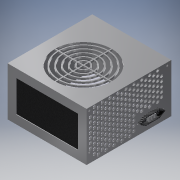
# Autodesk Inventor part: LC600H-12
Saved by Autodesk Inventor 2018.3 (Build 223284000, 284)
## iProperties
Created: 2019-03-04
Part Number: LC600H-12
Material: Generico
Document SubType Name: Modeling
Designer: AlfyPc
Density: 1 g/cm^3
Appearance: Alluminio - Scuro
Author: AlfyPc
Autodesk Inventor part; units mm, degrees
(part 1 of 4)
ref_plane "YZ Plane" through (0, 0, 0) normal (1, 0, 0) x (0, 1, 0)
ref_plane "XZ Plane" through (0, 0, 0) normal (0, 1, 0) x (-1, 0, 0)
ref_plane "XY Plane" through (0, 0, 0) normal (0, 0, 1) x (1, 0, 0)
sketch "Schizzo1" plane through (0, 0, 0) normal (0, 0, 1) x (1, 0, 0)
  line L0 (-70, 75) -> (70, 75)
  line L1 (70, 75) -> (70, -75)
  line L2 (70, -75) -> (-70, -75)
  line L3 (-70, -75) -> (-70, 75)
  line L4 (-70, 75) -> (70, -75) construction
  line L5 (70, 75) -> (-70, -75) construction
  line L6 (-70, 75) -> (70, 75) construction
  point P0 (0, 0)
  dimension "d0" = 140
  dimension "d1" = 0
  dimension "d2" = 150
  constraints: 14 end point, 2 horizontal, 2 midpoint, 2 parallel, 1 collinear, 1 perpendicular
  measures "d0" distance of L0.start L0.end
  measures "d1" distance between parallel lines of L0 L6
  measures "d2" distance of L0.end L1.end
extrude "Estrusione1" add sketch "Schizzo1" along normal blind 86
shell "Svuotamento1" thickness 3 removed faces 1 at (-23.3333, 25, 86)
sketch "Schizzo3" plane through (0, 0, 86) normal (0, 0, 1) x (1, 0, 0)
  line L0 (67, 72) -> (67, -72)
  line L1 (67, -72) -> (-67, -72)
  line L2 (-67, -72) -> (-67, 72)
  line L3 (-67, 72) -> (67, 72)
  line L4 (70, 75) -> (-70, 75)
  line L5 (-70, 75) -> (-70, -75)
  line L6 (-70, -75) -> (70, -75)
  line L7 (70, -75) -> (70, 75)
  line L8 (-1, 39.3407) -> (-1, 34.3396)
  line L9 (1, 34.3396) -> (1, 39.3407)
  line L10 (-1, 32.339) -> (-1, 25.837)
  line L11 (1, 25.837) -> (1, 32.339)
  line L12 (-1, 23.8362) -> (-1, 17.3328)
  line L13 (1, 17.3328) -> (1, 23.8362)
  line L14 (1, 0.3051) -> (1, 15.3314)
  line L15 (-1, 15.3314) -> (-1, 0.3051)
  line L16 (1, -28.1207) -> (1, -21.6038)
  line L17 (-1, -21.6038) -> (-1, -28.1207)
  line L18 (1, -36.6301) -> (1, -30.1237)
  line L19 (-1, -30.1237) -> (-1, -36.6301)
  line L20 (1, -45.1348) -> (1, -38.6315)
  line L21 (-1, -38.6315) -> (-1, -45.1348)
  line L22 (1, -60.6393) -> (1, -55.6382)
  line L23 (1, -53.6377) -> (1, -47.1356)
  line L24 (-1, -47.1356) -> (-1, -53.6377)
  line L25 (-1, -55.6382) -> (-1, -60.6393)
  line L26 (1, -19.5936) -> (1, -11.6493)
  line L27 (1, -9.6493) -> (1, -1.7051)
  line L28 (-1, -1.7051) -> (-1, -9.6493)
  line L29 (-1, -11.6493) -> (-1, -19.5936)
  line L30 (-8.9443, -9.6493) -> (-1, -9.6493)
  line L31 (-1, -11.6493) -> (-8.9443, -11.6493)
  line L32 (1, -9.6493) -> (8.9443, -9.6493)
  line L33 (8.9443, -11.6493) -> (1, -11.6493)
  line L34 (-17.4714, -9.6493) -> (-10.9545, -9.6493)
  line L35 (-10.9545, -11.6493) -> (-17.4714, -11.6493)
  line L36 (-49.99, -9.6493) -> (-27.9821, -9.6493)
  line L37 (-25.9808, -9.6493) -> (-19.4743, -9.6493)
  line L38 (-19.4743, -11.6493) -> (-25.9808, -11.6493)
  line L39 (-27.9821, -11.6493) -> (-49.99, -11.6493)
  line L40 (10.9545, -9.6493) -> (17.4714, -9.6493)
  line L41 (17.4714, -11.6493) -> (10.9545, -11.6493)
  arc A0 (1, -30.1237) -> (19.4743, -11.6493) centre (0, -10.6493) ccw
  arc A1 (19.4743, -9.6493) -> (1, 8.825) centre (0, -10.6493) ccw
  arc A2 (1, -28.1207) -> (17.4714, -11.6493) centre (0, -10.6493) ccw
  arc A3 (17.4714, -9.6493) -> (1, 6.8221) centre (0, -10.6493) ccw
  arc A4 (1, -21.6038) -> (10.9545, -11.6493) centre (0, -10.6493) ccw
  arc A5 (10.9545, -9.6493) -> (1, 0.3051) centre (0, -10.6493) ccw
  arc A6 (1, -19.5936) -> (8.9443, -11.6493) centre (0, -10.6493) ccw
  arc A7 (8.9443, -9.6493) -> (1, -1.7051) centre (0, -10.6493) ccw
  arc A8 (-1, -1.7051) -> (-8.9443, -9.6493) centre (0, -10.6493) ccw
  arc A9 (-8.9443, -11.6493) -> (-1, -19.5936) centre (0, -10.6493) ccw
  arc A10 (-1, 0.3051) -> (-10.9545, -9.6493) centre (0, -10.6493) ccw
  arc A11 (-10.9545, -11.6493) -> (-1, -21.6038) centre (0, -10.6493) ccw
  arc A12 (-1, 6.8221) -> (-17.4714, -9.6493) centre (0, -10.6493) ccw
  arc A13 (-17.4714, -11.6493) -> (-1, -28.1207) centre (0, -10.6493) ccw
  arc A14 (-1, 8.825) -> (-19.4743, -9.6493) centre (0, -10.6493) ccw
  arc A15 (-19.4743, -11.6493) -> (-1, -30.1237) centre (0, -10.6493) ccw
  arc A16 (-1, 15.3314) -> (-25.9808, -9.6493) centre (0, -10.6493) ccw
  arc A17 (-25.9808, -11.6493) -> (-1, -36.6301) centre (0, -10.6493) ccw
  arc A18 (-1, 17.3328) -> (-27.9821, -9.6493) centre (0, -10.6493) ccw
  arc A19 (-27.9821, -11.6493) -> (-1, -38.6315) centre (0, -10.6493) ccw
  arc A20 (-1, 23.8362) -> (-34.4855, -9.6493) centre (0, -10.6493) ccw
  arc A21 (-34.4855, -11.6493) -> (-1, -45.1348) centre (0, -10.6493) ccw
  arc A22 (-1, 25.837) -> (-36.4863, -9.6493) centre (0, -10.6493) ccw
  arc A23 (-36.4863, -11.6493) -> (-1, -47.1356) centre (0, -10.6493) ccw
  arc A24 (-1, 32.339) -> (-42.9884, -9.6493) centre (0, -10.6493) ccw
  arc A25 (-42.9884, -11.6493) -> (-1, -53.6377) centre (0, -10.6493) ccw
  arc A26 (-1, 34.3396) -> (-44.9889, -9.6493) centre (0, -10.6493) ccw
  arc A27 (-44.9889, -11.6493) -> (-1, -55.6382) centre (0, -10.6493) ccw
  arc A28 (-1, 39.3407) -> (-49.99, -9.6493) centre (0, -10.6493) ccw
  arc A29 (-49.99, -11.6493) -> (-1, -60.6393) centre (0, -10.6493) ccw
  arc A30 (1, -60.6393) -> (49.99, -11.6493) centre (0, -10.6493) ccw
  arc A31 (49.99, -9.6493) -> (1, 39.3407) centre (0, -10.6493) ccw
  arc A32 (1, -55.6382) -> (44.9889, -11.6493) centre (0, -10.6493) ccw
  arc A33 (44.9889, -9.6493) -> (1, 34.3396) centre (0, -10.6493) ccw
  arc A34 (1, -53.6377) -> (42.9884, -11.6493) centre (0, -10.6493) ccw
  arc A35 (42.9884, -9.6493) -> (1, 32.339) centre (0, -10.6493) ccw
  arc A36 (1, -47.1356) -> (36.4863, -11.6493) centre (0, -10.6493) ccw
  arc A37 (36.4863, -9.6493) -> (1, 25.837) centre (0, -10.6493) ccw
  arc A38 (1, -45.1348) -> (34.4855, -11.6493) centre (0, -10.6493) ccw
  arc A39 (34.4855, -9.6493) -> (1, 23.8362) centre (0, -10.6493) ccw
  arc A40 (1, -38.6315) -> (27.9821, -11.6493) centre (0, -10.6493) ccw
  arc A41 (27.9821, -9.6493) -> (1, 17.3328) centre (0, -10.6493) ccw
  arc A42 (1, -36.6301) -> (25.9808, -11.6493) centre (0, -10.6493) ccw
  arc A43 (25.9808, -9.6493) -> (1, 15.3314) centre (0, -10.6493) ccw
  line L42 (19.4743, -9.6493) -> (25.9808, -9.6493)
  line L43 (25.9808, -11.6493) -> (19.4743, -11.6493)
  line L44 (27.9821, -9.6493) -> (34.4855, -9.6493)
  line L45 (34.4855, -11.6493) -> (27.9821, -11.6493)
  line L46 (36.4863, -9.6493) -> (42.9884, -9.6493)
  line L47 (44.9889, -9.6493) -> (49.99, -9.6493)
  line L48 (49.99, -11.6493) -> (44.9889, -11.6493)
  line L49 (42.9884, -11.6493) -> (36.4863, -11.6493)
  point P0 (0, 0)
  constraints: 221 parallel, 84 end point, 12 point on line, 8 point on circle, 4 centre point, 121 other
extrude "Estrusione2" add sketch "Schizzo3" against normal blind 3 contours L0 L1 L2 L3
sketch "Schizzo4" plane through (70, -75, 0) normal (1, 0, 0) x (0, 0, -1)
  line L0 (-9, 7) -> (-7.5, 9.5981)
  line L1 (-7.5, 9.5981) -> (-4.5, 9.5981)
  line L2 (-4.5, 9.5981) -> (-3, 7)
  line L3 (-3, 7) -> (-4.5, 4.4019)
  line L4 (-4.5, 4.4019) -> (-7.5, 4.4019)
  line L5 (-7.5, 4.4019) -> (-9, 7)
  line L6 (-17, 7) -> (-15.5, 9.5981)
  line L7 (-15.5, 9.5981) -> (-12.5, 9.5981)
  line L8 (-12.5, 9.5981) -> (-11, 7)
  line L9 (-11, 7) -> (-12.5, 4.4019)
  line L10 (-12.5, 4.4019) -> (-15.5, 4.4019)
  line L11 (-15.5, 4.4019) -> (-17, 7)
  line L12 (-25, 7) -> (-23.5, 9.5981)
  line L13 (-23.5, 9.5981) -> (-20.5, 9.5981)
  line L14 (-20.5, 9.5981) -> (-19, 7)
  line L15 (-19, 7) -> (-20.5, 4.4019)
  line L16 (-20.5, 4.4019) -> (-23.5, 4.4019)
  line L17 (-23.5, 4.4019) -> (-25, 7)
  line L18 (-33, 7) -> (-31.5, 9.5981)
  line L19 (-31.5, 9.5981) -> (-28.5, 9.5981)
  line L20 (-28.5, 9.5981) -> (-27, 7)
  line L21 (-27, 7) -> (-28.5, 4.4019)
  line L22 (-28.5, 4.4019) -> (-31.5, 4.4019)
  line L23 (-31.5, 4.4019) -> (-33, 7)
  line L24 (-41, 7) -> (-39.5, 9.5981)
  line L25 (-39.5, 9.5981) -> (-36.5, 9.5981)
  line L26 (-36.5, 9.5981) -> (-35, 7)
  line L27 (-35, 7) -> (-36.5, 4.4019)
  line L28 (-36.5, 4.4019) -> (-39.5, 4.4019)
  line L29 (-39.5, 4.4019) -> (-41, 7)
  line L30 (-49, 7) -> (-47.5, 9.5981)
  line L31 (-47.5, 9.5981) -> (-44.5, 9.5981)
  line L32 (-44.5, 9.5981) -> (-43, 7)
  line L33 (-43, 7) -> (-44.5, 4.4019)
  line L34 (-44.5, 4.4019) -> (-47.5, 4.4019)
  line L35 (-47.5, 4.4019) -> (-49, 7)
  line L36 (-57, 7) -> (-55.5, 9.5981)
  line L37 (-55.5, 9.5981) -> (-52.5, 9.5981)
  line L38 (-52.5, 9.5981) -> (-51, 7)
  line L39 (-51, 7) -> (-52.5, 4.4019)
  line L40 (-52.5, 4.4019) -> (-55.5, 4.4019)
  line L41 (-55.5, 4.4019) -> (-57, 7)
  line L42 (-65, 7) -> (-63.5, 9.5981)
  line L43 (-63.5, 9.5981) -> (-60.5, 9.5981)
  line L44 (-60.5, 9.5981) -> (-59, 7)
  line L45 (-59, 7) -> (-60.5, 4.4019)
  line L46 (-60.5, 4.4019) -> (-63.5, 4.4019)
  line L47 (-63.5, 4.4019) -> (-65, 7)
  line L48 (-73, 7) -> (-71.5, 9.5981)
  line L49 (-71.5, 9.5981) -> (-68.5, 9.5981)
  line L50 (-68.5, 9.5981) -> (-67, 7)
  line L51 (-67, 7) -> (-68.5, 4.4019)
  line L52 (-68.5, 4.4019) -> (-71.5, 4.4019)
  line L53 (-71.5, 4.4019) -> (-73, 7)
  line L54 (-81, 7) -> (-79.5, 9.5981)
  line L55 (-79.5, 9.5981) -> (-76.5, 9.5981)
  line L56 (-76.5, 9.5981) -> (-75, 7)
  line L57 (-75, 7) -> (-76.5, 4.4019)
  line L58 (-76.5, 4.4019) -> (-79.5, 4.4019)
  line L59 (-79.5, 4.4019) -> (-81, 7)
  line L60 (-13, 13.9282) -> (-11.5, 16.5263)
  line L61 (-11.5, 16.5263) -> (-8.5, 16.5263)
  line L62 (-8.5, 16.5263) -> (-7, 13.9282)
  line L63 (-7, 13.9282) -> (-8.5, 11.3301)
  line L64 (-8.5, 11.3301) -> (-11.5, 11.3301)
  line L65 (-11.5, 11.3301) -> (-13, 13.9282)
  line L66 (-21, 13.9282) -> (-19.5, 16.5263)
  line L67 (-19.5, 16.5263) -> (-16.5, 16.5263)
  line L68 (-16.5, 16.5263) -> (-15, 13.9282)
  line L69 (-15, 13.9282) -> (-16.5, 11.3301)
  line L70 (-16.5, 11.3301) -> (-19.5, 11.3301)
  line L71 (-19.5, 11.3301) -> (-21, 13.9282)
  line L72 (-29, 13.9282) -> (-27.5, 16.5263)
  line L73 (-27.5, 16.5263) -> (-24.5, 16.5263)
  line L74 (-24.5, 16.5263) -> (-23, 13.9282)
  line L75 (-23, 13.9282) -> (-24.5, 11.3301)
  line L76 (-24.5, 11.3301) -> (-27.5, 11.3301)
  line L77 (-27.5, 11.3301) -> (-29, 13.9282)
  line L78 (-37, 13.9282) -> (-35.5, 16.5263)
  line L79 (-35.5, 16.5263) -> (-32.5, 16.5263)
  line L80 (-32.5, 16.5263) -> (-31, 13.9282)
  line L81 (-31, 13.9282) -> (-32.5, 11.3301)
  line L82 (-32.5, 11.3301) -> (-35.5, 11.3301)
  line L83 (-35.5, 11.3301) -> (-37, 13.9282)
  line L84 (-45, 13.9282) -> (-43.5, 16.5263)
  line L85 (-43.5, 16.5263) -> (-40.5, 16.5263)
  line L86 (-40.5, 16.5263) -> (-39, 13.9282)
  line L87 (-39, 13.9282) -> (-40.5, 11.3301)
  line L88 (-40.5, 11.3301) -> (-43.5, 11.3301)
  line L89 (-43.5, 11.3301) -> (-45, 13.9282)
  line L90 (-53, 13.9282) -> (-51.5, 16.5263)
  line L91 (-51.5, 16.5263) -> (-48.5, 16.5263)
  line L92 (-48.5, 16.5263) -> (-47, 13.9282)
  line L93 (-47, 13.9282) -> (-48.5, 11.3301)
  line L94 (-48.5, 11.3301) -> (-51.5, 11.3301)
  line L95 (-51.5, 11.3301) -> (-53, 13.9282)
  line L96 (-61, 13.9282) -> (-59.5, 16.5263)
  line L97 (-59.5, 16.5263) -> (-56.5, 16.5263)
  line L98 (-56.5, 16.5263) -> (-55, 13.9282)
  line L99 (-55, 13.9282) -> (-56.5, 11.3301)
  line L100 (-56.5, 11.3301) -> (-59.5, 11.3301)
  line L101 (-59.5, 11.3301) -> (-61, 13.9282)
  line L102 (-69, 13.9282) -> (-67.5, 16.5263)
  line L103 (-67.5, 16.5263) -> (-64.5, 16.5263)
  line L104 (-64.5, 16.5263) -> (-63, 13.9282)
  line L105 (-63, 13.9282) -> (-64.5, 11.3301)
  line L106 (-64.5, 11.3301) -> (-67.5, 11.3301)
  line L107 (-67.5, 11.3301) -> (-69, 13.9282)
  line L108 (-77, 13.9282) -> (-75.5, 16.5263)
  line L109 (-75.5, 16.5263) -> (-72.5, 16.5263)
  line L110 (-72.5, 16.5263) -> (-71, 13.9282)
  line L111 (-71, 13.9282) -> (-72.5, 11.3301)
  line L112 (-72.5, 11.3301) -> (-75.5, 11.3301)
  line L113 (-75.5, 11.3301) -> (-77, 13.9282)
  line L114 (-85, 13.9282) -> (-83.5, 16.5263)
  line L115 (-83.5, 16.5263) -> (-80.5, 16.5263)
  line L116 (-80.5, 16.5263) -> (-79, 13.9282)
  line L117 (-79, 13.9282) -> (-80.5, 11.3301)
  line L118 (-80.5, 11.3301) -> (-83.5, 11.3301)
  line L119 (-83.5, 11.3301) -> (-85, 13.9282)
  line L120 (-17, 20.8564) -> (-15.5, 23.4545)
  line L121 (-15.5, 23.4545) -> (-12.5, 23.4545)
  line L122 (-12.5, 23.4545) -> (-11, 20.8564)
  line L123 (-11, 20.8564) -> (-12.5, 18.2583)
  line L124 (-12.5, 18.2583) -> (-15.5, 18.2583)
  line L125 (-15.5, 18.2583) -> (-17, 20.8564)
  line L126 (-25, 20.8564) -> (-23.5, 23.4545)
  line L127 (-23.5, 23.4545) -> (-20.5, 23.4545)
  line L128 (-20.5, 23.4545) -> (-19, 20.8564)
  line L129 (-19, 20.8564) -> (-20.5, 18.2583)
  line L130 (-20.5, 18.2583) -> (-23.5, 18.2583)
  line L131 (-23.5, 18.2583) -> (-25, 20.8564)
  line L132 (-33, 20.8564) -> (-31.5, 23.4545)
  line L133 (-31.5, 23.4545) -> (-28.5, 23.4545)
  line L134 (-28.5, 23.4545) -> (-27, 20.8564)
  line L135 (-27, 20.8564) -> (-28.5, 18.2583)
  line L136 (-28.5, 18.2583) -> (-31.5, 18.2583)
  line L137 (-31.5, 18.2583) -> (-33, 20.8564)
  line L138 (-41, 20.8564) -> (-39.5, 23.4545)
  line L139 (-39.5, 23.4545) -> (-36.5, 23.4545)
  line L140 (-36.5, 23.4545) -> (-35, 20.8564)
  line L141 (-35, 20.8564) -> (-36.5, 18.2583)
  line L142 (-36.5, 18.2583) -> (-39.5, 18.2583)
  line L143 (-39.5, 18.2583) -> (-41, 20.8564)
  line L144 (-49, 20.8564) -> (-47.5, 23.4545)
  line L145 (-47.5, 23.4545) -> (-44.5, 23.4545)
  line L146 (-44.5, 23.4545) -> (-43, 20.8564)
  line L147 (-43, 20.8564) -> (-44.5, 18.2583)
  line L148 (-44.5, 18.2583) -> (-47.5, 18.2583)
  line L149 (-47.5, 18.2583) -> (-49, 20.8564)
  line L150 (-57, 20.8564) -> (-55.5, 23.4545)
  line L151 (-55.5, 23.4545) -> (-52.5, 23.4545)
  line L152 (-52.5, 23.4545) -> (-51, 20.8564)
  line L153 (-51, 20.8564) -> (-52.5, 18.2583)
  line L154 (-52.5, 18.2583) -> (-55.5, 18.2583)
  line L155 (-55.5, 18.2583) -> (-57, 20.8564)
  line L156 (-65, 20.8564) -> (-63.5, 23.4545)
  line L157 (-63.5, 23.4545) -> (-60.5, 23.4545)
  line L158 (-60.5, 23.4545) -> (-59, 20.8564)
  line L159 (-59, 20.8564) -> (-60.5, 18.2583)
  line L160 (-60.5, 18.2583) -> (-63.5, 18.2583)
  line L161 (-63.5, 18.2583) -> (-65, 20.8564)
  line L162 (-73, 20.8564) -> (-71.5, 23.4545)
  line L163 (-71.5, 23.4545) -> (-68.5, 23.4545)
  line L164 (-68.5, 23.4545) -> (-67, 20.8564)
  line L165 (-67, 20.8564) -> (-68.5, 18.2583)
  line L166 (-68.5, 18.2583) -> (-71.5, 18.2583)
  line L167 (-71.5, 18.2583) -> (-73, 20.8564)
  line L168 (-81, 20.8564) -> (-79.5, 23.4545)
  line L169 (-79.5, 23.4545) -> (-76.5, 23.4545)
  line L170 (-76.5, 23.4545) -> (-75, 20.8564)
  line L171 (-75, 20.8564) -> (-76.5, 18.2583)
  line L172 (-76.5, 18.2583) -> (-79.5, 18.2583)
  line L173 (-79.5, 18.2583) -> (-81, 20.8564)
  line L174 (-89, 20.8564) -> (-87.5, 23.4545)
  line L175 (-87.5, 23.4545) -> (-84.5, 23.4545)
  line L176 (-84.5, 23.4545) -> (-83, 20.8564)
  line L177 (-83, 20.8564) -> (-84.5, 18.2583)
  line L178 (-84.5, 18.2583) -> (-87.5, 18.2583)
  line L179 (-87.5, 18.2583) -> (-89, 20.8564)
  line L180 (-9, 20.8564) -> (-7.5, 23.4545)
  line L181 (-7.5, 18.2583) -> (-9, 20.8564)
  line L182 (-7.5, 23.4545) -> (-4.5, 23.4545)
  line L183 (-4.5, 18.2583) -> (-7.5, 18.2583)
  line L184 (-3, 20.8564) -> (-4.5, 18.2583)
  line L185 (-4.5, 23.4545) -> (-3, 20.8564)
  line L186 (-3, 7) -> (-3, 20.8564) construction
  line L187 (-80.5, 25.3301) -> (-83.5, 25.3301)
  line L188 (-83.5, 25.3301) -> (-85, 27.9282)
  line L189 (-85, 27.9282) -> (-83.5, 30.5263)
  line L190 (-83.5, 30.5263) -> (-80.5, 30.5263)
  line L191 (-72.5, 25.3301) -> (-75.5, 25.3301)
  line L192 (-75.5, 25.3301) -> (-77, 27.9282)
  line L193 (-80.5, 30.5263) -> (-79, 27.9282)
  line L194 (-77, 27.9282) -> (-75.5, 30.5263)
  line L195 (-71, 27.9282) -> (-72.5, 25.3301)
  line L196 (-75.5, 30.5263) -> (-72.5, 30.5263)
  line L197 (-72.5, 30.5263) -> (-71, 27.9282)
  line L198 (-79, 27.9282) -> (-80.5, 25.3301)
  line L199 (-51.5, 30.5263) -> (-48.5, 30.5263)
  line L200 (-48.5, 25.3301) -> (-51.5, 25.3301)
  line L201 (-51.5, 25.3301) -> (-53, 27.9282)
  line L202 (-53, 27.9282) -> (-51.5, 30.5263)
  line L203 (-56.5, 30.5263) -> (-55, 27.9282)
  line L204 (-55, 27.9282) -> (-56.5, 25.3301)
  line L205 (-56.5, 25.3301) -> (-59.5, 25.3301)
  line L206 (-59.5, 30.5263) -> (-56.5, 30.5263)
  line L207 (-61, 27.9282) -> (-59.5, 30.5263)
  line L208 (-64.5, 30.5263) -> (-63, 27.9282)
  line L209 (-63, 27.9282) -> (-64.5, 25.3301)
  line L210 (-67.5, 30.5263) -> (-64.5, 30.5263)
  line L211 (-64.5, 25.3301) -> (-67.5, 25.3301)
  line L212 (-69, 27.9282) -> (-67.5, 30.5263)
  line L213 (-67.5, 25.3301) -> (-69, 27.9282)
  line L214 (-59.5, 25.3301) -> (-61, 27.9282)
  line L215 (-76.5, 32.2583) -> (-79.5, 32.2583)
  line L216 (-79.5, 32.2583) -> (-81, 34.8564)
  line L217 (-79.5, 37.4545) -> (-76.5, 37.4545)
  line L218 (-81, 34.8564) -> (-79.5, 37.4545)
  line L219 (-39.5, 32.2583) -> (-41, 34.8564)
  line L220 (-41, 34.8564) -> (-39.5, 37.4545)
  line L221 (-43, 34.8564) -> (-44.5, 32.2583)
  line L222 (-44.5, 37.4545) -> (-43, 34.8564)
  line L223 (-47.5, 37.4545) -> (-44.5, 37.4545)
  line L224 (-49, 34.8564) -> (-47.5, 37.4545)
  line L225 (-47.5, 32.2583) -> (-49, 34.8564)
  line L226 (-52.5, 37.4545) -> (-51, 34.8564)
  line L227 (-51, 34.8564) -> (-52.5, 32.2583)
  line L228 (-55.5, 37.4545) -> (-52.5, 37.4545)
  line L229 (-52.5, 32.2583) -> (-55.5, 32.2583)
  line L230 (-44.5, 32.2583) -> (-47.5, 32.2583)
  line L231 (-57, 34.8564) -> (-55.5, 37.4545)
  line L232 (-60.5, 37.4545) -> (-59, 34.8564)
  line L233 (-59, 34.8564) -> (-60.5, 32.2583)
  line L234 (-63.5, 37.4545) -> (-60.5, 37.4545)
  line L235 (-60.5, 32.2583) -> (-63.5, 32.2583)
  line L236 (-63.5, 32.2583) -> (-65, 34.8564)
  line L237 (-65, 34.8564) -> (-63.5, 37.4545)
  line L238 (-55.5, 32.2583) -> (-57, 34.8564)
  line L239 (-67, 34.8564) -> (-68.5, 32.2583)
  line L240 (-68.5, 37.4545) -> (-67, 34.8564)
  line L241 (-68.5, 32.2583) -> (-71.5, 32.2583)
  line L242 (-71.5, 32.2583) -> (-73, 34.8564)
  line L243 (-73, 34.8564) -> (-71.5, 37.4545)
  line L244 (-75, 34.8564) -> (-76.5, 32.2583)
  line L245 (-76.5, 37.4545) -> (-75, 34.8564)
  line L246 (-71.5, 37.4545) -> (-68.5, 37.4545)
  line L247 (-47, 27.9282) -> (-48.5, 25.3301)
  line L248 (-48.5, 30.5263) -> (-47, 27.9282)
  line L249 (-45, 27.9282) -> (-43.5, 30.5263)
  line L250 (-43.5, 25.3301) -> (-45, 27.9282)
  line L251 (-43.5, 30.5263) -> (-40.5, 30.5263)
  line L252 (-40.5, 25.3301) -> (-43.5, 25.3301)
  line L253 (-40.5, 30.5263) -> (-39, 27.9282)
  line L254 (-39, 27.9282) -> (-40.5, 25.3301)
  line L255 (-11, 34.8564) -> (-12.5, 32.2583)
  line L256 (-12.5, 37.4545) -> (-11, 34.8564)
  line L257 (-24.5, 30.5263) -> (-23, 27.9282)
  line L258 (-23, 27.9282) -> (-24.5, 25.3301)
  line L259 (-27.5, 30.5263) -> (-24.5, 30.5263)
  line L260 (-24.5, 25.3301) -> (-27.5, 25.3301)
  line L261 (-29, 27.9282) -> (-27.5, 30.5263)
  line L262 (-27.5, 25.3301) -> (-29, 27.9282)
  line L263 (-31, 27.9282) -> (-32.5, 25.3301)
  line L264 (-32.5, 30.5263) -> (-31, 27.9282)
  line L265 (-32.5, 25.3301) -> (-35.5, 25.3301)
  line L266 (-35.5, 30.5263) -> (-32.5, 30.5263)
  line L267 (-35.5, 25.3301) -> (-37, 27.9282)
  line L268 (-37, 27.9282) -> (-35.5, 30.5263)
  line L269 (-19.5, 25.3301) -> (-21, 27.9282)
  line L270 (-21, 27.9282) -> (-19.5, 30.5263)
  line L271 (-19.5, 30.5263) -> (-16.5, 30.5263)
  line L272 (-16.5, 25.3301) -> (-19.5, 25.3301)
  line L273 (-16.5, 30.5263) -> (-15, 27.9282)
  line L274 (-15, 27.9282) -> (-16.5, 25.3301)
  line L275 (-20.5, 32.2583) -> (-23.5, 32.2583)
  line L276 (-23.5, 37.4545) -> (-20.5, 37.4545)
  line L277 (-19, 34.8564) -> (-20.5, 32.2583)
  line L278 (-20.5, 37.4545) -> (-19, 34.8564)
  line L279 (-17, 34.8564) -> (-15.5, 37.4545)
  line L280 (-15.5, 32.2583) -> (-17, 34.8564)
  line L281 (-12.5, 32.2583) -> (-15.5, 32.2583)
  line L282 (-15.5, 37.4545) -> (-12.5, 37.4545)
  line L283 (-25, 34.8564) -> (-23.5, 37.4545)
  line L284 (-28.5, 37.4545) -> (-27, 34.8564)
  line L285 (-27, 34.8564) -> (-28.5, 32.2583)
  line L286 (-31.5, 37.4545) -> (-28.5, 37.4545)
  line L287 (-28.5, 32.2583) -> (-31.5, 32.2583)
  line L288 (-33, 34.8564) -> (-31.5, 37.4545)
  line L289 (-31.5, 32.2583) -> (-33, 34.8564)
  line L290 (-23.5, 32.2583) -> (-25, 34.8564)
  line L291 (-36.5, 37.4545) -> (-35, 34.8564)
  line L292 (-35, 34.8564) -> (-36.5, 32.2583)
  line L293 (-39.5, 37.4545) -> (-36.5, 37.4545)
  line L294 (-36.5, 32.2583) -> (-39.5, 32.2583)
  line L295 (-13, 27.9282) -> (-11.5, 30.5263)
  line L296 (-8.5, 25.3301) -> (-11.5, 25.3301)
  line L297 (-11.5, 25.3301) -> (-13, 27.9282)
  line L298 (-8.5, 30.5263) -> (-7, 27.9282)
  line L299 (-7, 27.9282) -> (-8.5, 25.3301)
  line L300 (-4.5, 32.2583) -> (-7.5, 32.2583)
  line L301 (-7.5, 32.2583) -> (-9, 34.8564)
  line L302 (-3, 34.8564) -> (-4.5, 32.2583)
  line L303 (-4.5, 37.4545) -> (-3, 34.8564)
  line L304 (-7.5, 37.4545) -> (-4.5, 37.4545)
  line L305 (-9, 34.8564) -> (-7.5, 37.4545)
  line L306 (-11.5, 30.5263) -> (-8.5, 30.5263)
  line L307 (-3, 21) -> (-3, 34.8564) construction
  line L308 (-80.5, 39.3301) -> (-83.5, 39.3301)
  line L309 (-83.5, 39.3301) -> (-85, 41.9282)
  line L310 (-85, 41.9282) -> (-83.5, 44.5263)
  line L311 (-83.5, 44.5263) -> (-80.5, 44.5263)
  line L312 (-72.5, 39.3301) -> (-75.5, 39.3301)
  line L313 (-75.5, 39.3301) -> (-77, 41.9282)
  line L314 (-80.5, 44.5263) -> (-79, 41.9282)
  line L315 (-77, 41.9282) -> (-75.5, 44.5263)
  line L316 (-71, 41.9282) -> (-72.5, 39.3301)
  line L317 (-75.5, 44.5263) -> (-72.5, 44.5263)
  line L318 (-72.5, 44.5263) -> (-71, 41.9282)
  line L319 (-79, 41.9282) -> (-80.5, 39.3301)
  line L320 (-51.5, 44.5263) -> (-48.5, 44.5263)
  line L321 (-48.5, 39.3301) -> (-51.5, 39.3301)
  line L322 (-51.5, 39.3301) -> (-53, 41.9282)
  line L323 (-53, 41.9282) -> (-51.5, 44.5263)
  line L324 (-56.5, 44.5263) -> (-55, 41.9282)
  line L325 (-55, 41.9282) -> (-56.5, 39.3301)
  line L326 (-56.5, 39.3301) -> (-59.5, 39.3301)
  line L327 (-59.5, 44.5263) -> (-56.5, 44.5263)
  line L328 (-61, 41.9282) -> (-59.5, 44.5263)
  line L329 (-64.5, 44.5263) -> (-63, 41.9282)
  line L330 (-63, 41.9282) -> (-64.5, 39.3301)
  line L331 (-67.5, 44.5263) -> (-64.5, 44.5263)
  line L332 (-64.5, 39.3301) -> (-67.5, 39.3301)
  line L333 (-69, 41.9282) -> (-67.5, 44.5263)
  line L334 (-67.5, 39.3301) -> (-69, 41.9282)
  line L335 (-59.5, 39.3301) -> (-61, 41.9282)
  line L336 (-76.5, 46.2583) -> (-79.5, 46.2583)
  line L337 (-79.5, 46.2583) -> (-81, 48.8564)
  line L338 (-79.5, 51.4545) -> (-76.5, 51.4545)
  line L339 (-81, 48.8564) -> (-79.5, 51.4545)
  line L340 (-39.5, 46.2583) -> (-41, 48.8564)
  line L341 (-41, 48.8564) -> (-39.5, 51.4545)
  line L342 (-43, 48.8564) -> (-44.5, 46.2583)
  line L343 (-44.5, 51.4545) -> (-43, 48.8564)
  line L344 (-47.5, 51.4545) -> (-44.5, 51.4545)
  line L345 (-49, 48.8564) -> (-47.5, 51.4545)
  line L346 (-47.5, 46.2583) -> (-49, 48.8564)
  line L347 (-52.5, 51.4545) -> (-51, 48.8564)
  line L348 (-51, 48.8564) -> (-52.5, 46.2583)
  line L349 (-55.5, 51.4545) -> (-52.5, 51.4545)
  line L350 (-52.5, 46.2583) -> (-55.5, 46.2583)
  line L351 (-44.5, 46.2583) -> (-47.5, 46.2583)
  line L352 (-57, 48.8564) -> (-55.5, 51.4545)
  line L353 (-60.5, 51.4545) -> (-59, 48.8564)
  line L354 (-59, 48.8564) -> (-60.5, 46.2583)
  line L355 (-63.5, 51.4545) -> (-60.5, 51.4545)
  line L356 (-60.5, 46.2583) -> (-63.5, 46.2583)
  line L357 (-63.5, 46.2583) -> (-65, 48.8564)
  line L358 (-65, 48.8564) -> (-63.5, 51.4545)
  line L359 (-55.5, 46.2583) -> (-57, 48.8564)
  line L360 (-67, 48.8564) -> (-68.5, 46.2583)
  line L361 (-68.5, 51.4545) -> (-67, 48.8564)
  line L362 (-68.5, 46.2583) -> (-71.5, 46.2583)
  line L363 (-71.5, 46.2583) -> (-73, 48.8564)
  line L364 (-73, 48.8564) -> (-71.5, 51.4545)
  line L365 (-75, 48.8564) -> (-76.5, 46.2583)
  line L366 (-76.5, 51.4545) -> (-75, 48.8564)
  line L367 (-71.5, 51.4545) -> (-68.5, 51.4545)
  line L368 (-47, 41.9282) -> (-48.5, 39.3301)
  line L369 (-48.5, 44.5263) -> (-47, 41.9282)
  line L370 (-45, 41.9282) -> (-43.5, 44.5263)
  line L371 (-43.5, 39.3301) -> (-45, 41.9282)
  line L372 (-43.5, 44.5263) -> (-40.5, 44.5263)
  line L373 (-40.5, 39.3301) -> (-43.5, 39.3301)
  line L374 (-40.5, 44.5263) -> (-39, 41.9282)
  line L375 (-39, 41.9282) -> (-40.5, 39.3301)
  line L376 (-11, 48.8564) -> (-12.5, 46.2583)
  line L377 (-12.5, 51.4545) -> (-11, 48.8564)
  line L378 (-24.5, 44.5263) -> (-23, 41.9282)
  line L379 (-23, 41.9282) -> (-24.5, 39.3301)
  line L380 (-27.5, 44.5263) -> (-24.5, 44.5263)
  line L381 (-24.5, 39.3301) -> (-27.5, 39.3301)
  line L382 (-29, 41.9282) -> (-27.5, 44.5263)
  line L383 (-27.5, 39.3301) -> (-29, 41.9282)
  line L384 (-31, 41.9282) -> (-32.5, 39.3301)
  line L385 (-32.5, 44.5263) -> (-31, 41.9282)
  line L386 (-32.5, 39.3301) -> (-35.5, 39.3301)
  line L387 (-35.5, 44.5263) -> (-32.5, 44.5263)
  line L388 (-35.5, 39.3301) -> (-37, 41.9282)
  line L389 (-37, 41.9282) -> (-35.5, 44.5263)
  line L390 (-19.5, 39.3301) -> (-21, 41.9282)
  line L391 (-21, 41.9282) -> (-19.5, 44.5263)
  line L392 (-19.5, 44.5263) -> (-16.5, 44.5263)
  line L393 (-16.5, 39.3301) -> (-19.5, 39.3301)
  line L394 (-16.5, 44.5263) -> (-15, 41.9282)
  line L395 (-15, 41.9282) -> (-16.5, 39.3301)
  line L396 (-20.5, 46.2583) -> (-23.5, 46.2583)
  line L397 (-23.5, 51.4545) -> (-20.5, 51.4545)
  line L398 (-19, 48.8564) -> (-20.5, 46.2583)
  line L399 (-20.5, 51.4545) -> (-19, 48.8564)
  line L400 (-17, 48.8564) -> (-15.5, 51.4545)
  line L401 (-15.5, 46.2583) -> (-17, 48.8564)
  line L402 (-12.5, 46.2583) -> (-15.5, 46.2583)
  line L403 (-15.5, 51.4545) -> (-12.5, 51.4545)
  line L404 (-25, 48.8564) -> (-23.5, 51.4545)
  line L405 (-28.5, 51.4545) -> (-27, 48.8564)
  line L406 (-27, 48.8564) -> (-28.5, 46.2583)
  line L407 (-31.5, 51.4545) -> (-28.5, 51.4545)
  line L408 (-28.5, 46.2583) -> (-31.5, 46.2583)
  line L409 (-33, 48.8564) -> (-31.5, 51.4545)
  line L410 (-31.5, 46.2583) -> (-33, 48.8564)
  line L411 (-23.5, 46.2583) -> (-25, 48.8564)
  line L412 (-36.5, 51.4545) -> (-35, 48.8564)
  line L413 (-35, 48.8564) -> (-36.5, 46.2583)
  line L414 (-39.5, 51.4545) -> (-36.5, 51.4545)
  line L415 (-36.5, 46.2583) -> (-39.5, 46.2583)
  line L416 (-13, 41.9282) -> (-11.5, 44.5263)
  line L417 (-8.5, 39.3301) -> (-11.5, 39.3301)
  line L418 (-11.5, 39.3301) -> (-13, 41.9282)
  line L419 (-8.5, 44.5263) -> (-7, 41.9282)
  line L420 (-7, 41.9282) -> (-8.5, 39.3301)
  line L421 (-4.5, 46.2583) -> (-7.5, 46.2583)
  line L422 (-7.5, 46.2583) -> (-9, 48.8564)
  line L423 (-3, 48.8564) -> (-4.5, 46.2583)
  line L424 (-4.5, 51.4545) -> (-3, 48.8564)
  line L425 (-7.5, 51.4545) -> (-4.5, 51.4545)
  line L426 (-9, 48.8564) -> (-7.5, 51.4545)
  line L427 (-11.5, 44.5263) -> (-8.5, 44.5263)
  line L428 (-3, 35) -> (-3, 48.8564) construction
  line L429 (-80.5, 53.3301) -> (-83.5, 53.3301)
  line L430 (-83.5, 53.3301) -> (-85, 55.9282)
  line L431 (-85, 55.9282) -> (-83.5, 58.5263)
  line L432 (-83.5, 58.5263) -> (-80.5, 58.5263)
  line L433 (-72.5, 53.3301) -> (-75.5, 53.3301)
  line L434 (-75.5, 53.3301) -> (-77, 55.9282)
  line L435 (-80.5, 58.5263) -> (-79, 55.9282)
  line L436 (-77, 55.9282) -> (-75.5, 58.5263)
  line L437 (-71, 55.9282) -> (-72.5, 53.3301)
  line L438 (-75.5, 58.5263) -> (-72.5, 58.5263)
  line L439 (-72.5, 58.5263) -> (-71, 55.9282)
  line L440 (-79, 55.9282) -> (-80.5, 53.3301)
  line L441 (-51.5, 58.5263) -> (-48.5, 58.5263)
  line L442 (-48.5, 53.3301) -> (-51.5, 53.3301)
  line L443 (-51.5, 53.3301) -> (-53, 55.9282)
  line L444 (-53, 55.9282) -> (-51.5, 58.5263)
  line L445 (-56.5, 58.5263) -> (-55, 55.9282)
  line L446 (-55, 55.9282) -> (-56.5, 53.3301)
  line L447 (-56.5, 53.3301) -> (-59.5, 53.3301)
  line L448 (-59.5, 58.5263) -> (-56.5, 58.5263)
  line L449 (-61, 55.9282) -> (-59.5, 58.5263)
  line L450 (-64.5, 58.5263) -> (-63, 55.9282)
  line L451 (-63, 55.9282) -> (-64.5, 53.3301)
  line L452 (-67.5, 58.5263) -> (-64.5, 58.5263)
  line L453 (-64.5, 53.3301) -> (-67.5, 53.3301)
  line L454 (-69, 55.9282) -> (-67.5, 58.5263)
  line L455 (-67.5, 53.3301) -> (-69, 55.9282)
  line L456 (-59.5, 53.3301) -> (-61, 55.9282)
  line L457 (-76.5, 60.2583) -> (-79.5, 60.2583)
  line L458 (-79.5, 60.2583) -> (-81, 62.8564)
  line L459 (-79.5, 65.4545) -> (-76.5, 65.4545)
  line L460 (-81, 62.8564) -> (-79.5, 65.4545)
  line L461 (-39.5, 60.2583) -> (-41, 62.8564)
  line L462 (-41, 62.8564) -> (-39.5, 65.4545)
  line L463 (-43, 62.8564) -> (-44.5, 60.2583)
  line L464 (-44.5, 65.4545) -> (-43, 62.8564)
  line L465 (-47.5, 65.4545) -> (-44.5, 65.4545)
  line L466 (-49, 62.8564) -> (-47.5, 65.4545)
  line L467 (-47.5, 60.2583) -> (-49, 62.8564)
  line L468 (-52.5, 65.4545) -> (-51, 62.8564)
  line L469 (-51, 62.8564) -> (-52.5, 60.2583)
  line L470 (-55.5, 65.4545) -> (-52.5, 65.4545)
  line L471 (-52.5, 60.2583) -> (-55.5, 60.2583)
  line L472 (-44.5, 60.2583) -> (-47.5, 60.2583)
  line L473 (-57, 62.8564) -> (-55.5, 65.4545)
  line L474 (-60.5, 65.4545) -> (-59, 62.8564)
  line L475 (-59, 62.8564) -> (-60.5, 60.2583)
  line L476 (-63.5, 65.4545) -> (-60.5, 65.4545)
  line L477 (-60.5, 60.2583) -> (-63.5, 60.2583)
  line L478 (-63.5, 60.2583) -> (-65, 62.8564)
  line L479 (-65, 62.8564) -> (-63.5, 65.4545)
  line L480 (-55.5, 60.2583) -> (-57, 62.8564)
  line L481 (-67, 62.8564) -> (-68.5, 60.2583)
  line L482 (-68.5, 65.4545) -> (-67, 62.8564)
  line L483 (-68.5, 60.2583) -> (-71.5, 60.2583)
  line L484 (-71.5, 60.2583) -> (-73, 62.8564)
  line L485 (-73, 62.8564) -> (-71.5, 65.4545)
  line L486 (-75, 62.8564) -> (-76.5, 60.2583)
  line L487 (-76.5, 65.4545) -> (-75, 62.8564)
  line L488 (-71.5, 65.4545) -> (-68.5, 65.4545)
  line L489 (-47, 55.9282) -> (-48.5, 53.3301)
  line L490 (-48.5, 58.5263) -> (-47, 55.9282)
  line L491 (-45, 55.9282) -> (-43.5, 58.5263)
  line L492 (-43.5, 53.3301) -> (-45, 55.9282)
  line L493 (-43.5, 58.5263) -> (-40.5, 58.5263)
  line L494 (-40.5, 53.3301) -> (-43.5, 53.3301)
  line L495 (-40.5, 58.5263) -> (-39, 55.9282)
  line L496 (-39, 55.9282) -> (-40.5, 53.3301)
  line L497 (-11, 62.8564) -> (-12.5, 60.2583)
  line L498 (-12.5, 65.4545) -> (-11, 62.8564)
  line L499 (-24.5, 58.5263) -> (-23, 55.9282)
  line L500 (-23, 55.9282) -> (-24.5, 53.3301)
  line L501 (-27.5, 58.5263) -> (-24.5, 58.5263)
  line L502 (-24.5, 53.3301) -> (-27.5, 53.3301)
  line L503 (-29, 55.9282) -> (-27.5, 58.5263)
  line L504 (-27.5, 53.3301) -> (-29, 55.9282)
  line L505 (-31, 55.9282) -> (-32.5, 53.3301)
  line L506 (-32.5, 58.5263) -> (-31, 55.9282)
  line L507 (-32.5, 53.3301) -> (-35.5, 53.3301)
  line L508 (-35.5, 58.5263) -> (-32.5, 58.5263)
  line L509 (-35.5, 53.3301) -> (-37, 55.9282)
  line L510 (-37, 55.9282) -> (-35.5, 58.5263)
  line L511 (-19.5, 53.3301) -> (-21, 55.9282)
  line L512 (-21, 55.9282) -> (-19.5, 58.5263)
  line L513 (-19.5, 58.5263) -> (-16.5, 58.5263)
  line L514 (-16.5, 53.3301) -> (-19.5, 53.3301)
  line L515 (-16.5, 58.5263) -> (-15, 55.9282)
  line L516 (-15, 55.9282) -> (-16.5, 53.3301)
  line L517 (-20.5, 60.2583) -> (-23.5, 60.2583)
  line L518 (-23.5, 65.4545) -> (-20.5, 65.4545)
  line L519 (-19, 62.8564) -> (-20.5, 60.2583)
  line L520 (-20.5, 65.4545) -> (-19, 62.8564)
  line L521 (-17, 62.8564) -> (-15.5, 65.4545)
  line L522 (-15.5, 60.2583) -> (-17, 62.8564)
  line L523 (-12.5, 60.2583) -> (-15.5, 60.2583)
  line L524 (-15.5, 65.4545) -> (-12.5, 65.4545)
  line L525 (-25, 62.8564) -> (-23.5, 65.4545)
  line L526 (-28.5, 65.4545) -> (-27, 62.8564)
  line L527 (-27, 62.8564) -> (-28.5, 60.2583)
  line L528 (-31.5, 65.4545) -> (-28.5, 65.4545)
  line L529 (-28.5, 60.2583) -> (-31.5, 60.2583)
  line L530 (-33, 62.8564) -> (-31.5, 65.4545)
  line L531 (-31.5, 60.2583) -> (-33, 62.8564)
  line L532 (-23.5, 60.2583) -> (-25, 62.8564)
  line L533 (-36.5, 65.4545) -> (-35, 62.8564)
  line L534 (-35, 62.8564) -> (-36.5, 60.2583)
  line L535 (-39.5, 65.4545) -> (-36.5, 65.4545)
  line L536 (-36.5, 60.2583) -> (-39.5, 60.2583)
  line L537 (-13, 55.9282) -> (-11.5, 58.5263)
  line L538 (-8.5, 53.3301) -> (-11.5, 53.3301)
  line L539 (-11.5, 53.3301) -> (-13, 55.9282)
  line L540 (-8.5, 58.5263) -> (-7, 55.9282)
  line L541 (-7, 55.9282) -> (-8.5, 53.3301)
  line L542 (-4.5, 60.2583) -> (-7.5, 60.2583)
  line L543 (-7.5, 60.2583) -> (-9, 62.8564)
  line L544 (-3, 62.8564) -> (-4.5, 60.2583)
  line L545 (-4.5, 65.4545) -> (-3, 62.8564)
  line L546 (-7.5, 65.4545) -> (-4.5, 65.4545)
  line L547 (-9, 62.8564) -> (-7.5, 65.4545)
  line L548 (-11.5, 58.5263) -> (-8.5, 58.5263)
  line L549 (-3, 49) -> (-3, 62.8564) construction
  line L550 (-80.5, 67.3301) -> (-83.5, 67.3301)
  line L551 (-83.5, 67.3301) -> (-85, 69.9282)
  line L552 (-85, 69.9282) -> (-83.5, 72.5263)
  line L553 (-83.5, 72.5263) -> (-80.5, 72.5263)
  line L554 (-72.5, 67.3301) -> (-75.5, 67.3301)
  line L555 (-75.5, 67.3301) -> (-77, 69.9282)
  line L556 (-80.5, 72.5263) -> (-79, 69.9282)
  line L557 (-77, 69.9282) -> (-75.5, 72.5263)
  line L558 (-71, 69.9282) -> (-72.5, 67.3301)
  line L559 (-75.5, 72.5263) -> (-72.5, 72.5263)
  line L560 (-72.5, 72.5263) -> (-71, 69.9282)
  line L561 (-79, 69.9282) -> (-80.5, 67.3301)
  line L562 (-51.5, 72.5263) -> (-48.5, 72.5263)
  line L563 (-48.5, 67.3301) -> (-51.5, 67.3301)
  line L564 (-51.5, 67.3301) -> (-53, 69.9282)
  line L565 (-53, 69.9282) -> (-51.5, 72.5263)
  line L566 (-56.5, 72.5263) -> (-55, 69.9282)
  line L567 (-55, 69.9282) -> (-56.5, 67.3301)
  line L568 (-56.5, 67.3301) -> (-59.5, 67.3301)
  line L569 (-59.5, 72.5263) -> (-56.5, 72.5263)
  line L570 (-61, 69.9282) -> (-59.5, 72.5263)
  line L571 (-64.5, 72.5263) -> (-63, 69.9282)
  line L572 (-63, 69.9282) -> (-64.5, 67.3301)
  line L573 (-67.5, 72.5263) -> (-64.5, 72.5263)
  line L574 (-64.5, 67.3301) -> (-67.5, 67.3301)
  line L575 (-69, 69.9282) -> (-67.5, 72.5263)
  line L576 (-67.5, 67.3301) -> (-69, 69.9282)
  line L577 (-59.5, 67.3301) -> (-61, 69.9282)
  line L578 (-76.5, 74.2583) -> (-79.5, 74.2583)
  line L579 (-79.5, 74.2583) -> (-81, 76.8564)
  line L580 (-79.5, 79.4545) -> (-76.5, 79.4545)
  line L581 (-81, 76.8564) -> (-79.5, 79.4545)
  line L582 (-39.5, 74.2583) -> (-41, 76.8564)
  line L583 (-41, 76.8564) -> (-39.5, 79.4545)
  line L584 (-43, 76.8564) -> (-44.5, 74.2583)
  line L585 (-44.5, 79.4545) -> (-43, 76.8564)
  line L586 (-47.5, 79.4545) -> (-44.5, 79.4545)
  line L587 (-49, 76.8564) -> (-47.5, 79.4545)
  line L588 (-47.5, 74.2583) -> (-49, 76.8564)
  line L589 (-52.5, 79.4545) -> (-51, 76.8564)
  line L590 (-51, 76.8564) -> (-52.5, 74.2583)
  line L591 (-55.5, 79.4545) -> (-52.5, 79.4545)
  line L592 (-52.5, 74.2583) -> (-55.5, 74.2583)
  line L593 (-44.5, 74.2583) -> (-47.5, 74.2583)
  line L594 (-57, 76.8564) -> (-55.5, 79.4545)
  line L595 (-60.5, 79.4545) -> (-59, 76.8564)
  line L596 (-59, 76.8564) -> (-60.5, 74.2583)
  line L597 (-63.5, 79.4545) -> (-60.5, 79.4545)
  line L598 (-60.5, 74.2583) -> (-63.5, 74.2583)
  line L599 (-63.5, 74.2583) -> (-65, 76.8564)
  line L600 (-65, 76.8564) -> (-63.5, 79.4545)
  line L601 (-55.5, 74.2583) -> (-57, 76.8564)
  line L602 (-67, 76.8564) -> (-68.5, 74.2583)
  line L603 (-68.5, 79.4545) -> (-67, 76.8564)
  line L604 (-68.5, 74.2583) -> (-71.5, 74.2583)
  line L605 (-71.5, 74.2583) -> (-73, 76.8564)
  line L606 (-73, 76.8564) -> (-71.5, 79.4545)
  line L607 (-75, 76.8564) -> (-76.5, 74.2583)
  line L608 (-76.5, 79.4545) -> (-75, 76.8564)
  line L609 (-71.5, 79.4545) -> (-68.5, 79.4545)
  line L610 (-47, 69.9282) -> (-48.5, 67.3301)
  line L611 (-48.5, 72.5263) -> (-47, 69.9282)
  line L612 (-45, 69.9282) -> (-43.5, 72.5263)
  line L613 (-43.5, 67.3301) -> (-45, 69.9282)
  line L614 (-43.5, 72.5263) -> (-40.5, 72.5263)
  line L615 (-40.5, 67.3301) -> (-43.5, 67.3301)
  line L616 (-40.5, 72.5263) -> (-39, 69.9282)
  line L617 (-39, 69.9282) -> (-40.5, 67.3301)
  line L618 (-11, 76.8564) -> (-12.5, 74.2583)
  line L619 (-12.5, 79.4545) -> (-11, 76.8564)
  line L620 (-24.5, 72.5263) -> (-23, 69.9282)
  line L621 (-23, 69.9282) -> (-24.5, 67.3301)
  line L622 (-27.5, 72.5263) -> (-24.5, 72.5263)
  line L623 (-24.5, 67.3301) -> (-27.5, 67.3301)
  line L624 (-29, 69.9282) -> (-27.5, 72.5263)
  line L625 (-27.5, 67.3301) -> (-29, 69.9282)
  line L626 (-31, 69.9282) -> (-32.5, 67.3301)
  line L627 (-32.5, 72.5263) -> (-31, 69.9282)
  line L628 (-32.5, 67.3301) -> (-35.5, 67.3301)
  line L629 (-35.5, 72.5263) -> (-32.5, 72.5263)
  line L630 (-35.5, 67.3301) -> (-37, 69.9282)
  line L631 (-37, 69.9282) -> (-35.5, 72.5263)
  line L632 (-19.5, 67.3301) -> (-21, 69.9282)
  line L633 (-21, 69.9282) -> (-19.5, 72.5263)
  line L634 (-19.5, 72.5263) -> (-16.5, 72.5263)
  line L635 (-16.5, 67.3301) -> (-19.5, 67.3301)
  line L636 (-16.5, 72.5263) -> (-15, 69.9282)
  line L637 (-15, 69.9282) -> (-16.5, 67.3301)
  line L638 (-20.5, 74.2583) -> (-23.5, 74.2583)
  line L639 (-23.5, 79.4545) -> (-20.5, 79.4545)
  line L640 (-19, 76.8564) -> (-20.5, 74.2583)
  line L641 (-20.5, 79.4545) -> (-19, 76.8564)
  line L642 (-17, 76.8564) -> (-15.5, 79.4545)
  line L643 (-15.5, 74.2583) -> (-17, 76.8564)
  line L644 (-12.5, 74.2583) -> (-15.5, 74.2583)
  line L645 (-15.5, 79.4545) -> (-12.5, 79.4545)
  line L646 (-25, 76.8564) -> (-23.5, 79.4545)
  line L647 (-28.5, 79.4545) -> (-27, 76.8564)
  line L648 (-27, 76.8564) -> (-28.5, 74.2583)
  line L649 (-31.5, 79.4545) -> (-28.5, 79.4545)
  line L650 (-28.5, 74.2583) -> (-31.5, 74.2583)
  line L651 (-33, 76.8564) -> (-31.5, 79.4545)
  line L652 (-31.5, 74.2583) -> (-33, 76.8564)
  line L653 (-23.5, 74.2583) -> (-25, 76.8564)
  line L654 (-36.5, 79.4545) -> (-35, 76.8564)
  line L655 (-35, 76.8564) -> (-36.5, 74.2583)
  line L656 (-39.5, 79.4545) -> (-36.5, 79.4545)
  line L657 (-36.5, 74.2583) -> (-39.5, 74.2583)
  line L658 (-13, 69.9282) -> (-11.5, 72.5263)
  line L659 (-8.5, 67.3301) -> (-11.5, 67.3301)
  line L660 (-11.5, 67.3301) -> (-13, 69.9282)
  line L661 (-8.5, 72.5263) -> (-7, 69.9282)
  line L662 (-7, 69.9282) -> (-8.5, 67.3301)
  line L663 (-4.5, 74.2583) -> (-7.5, 74.2583)
  line L664 (-7.5, 74.2583) -> (-9, 76.8564)
  line L665 (-3, 76.8564) -> (-4.5, 74.2583)
  line L666 (-4.5, 79.4545) -> (-3, 76.8564)
  line L667 (-7.5, 79.4545) -> (-4.5, 79.4545)
  line L668 (-9, 76.8564) -> (-7.5, 79.4545)
  line L669 (-11.5, 72.5263) -> (-8.5, 72.5263)
  line L670 (-3, 63) -> (-3, 76.8564) construction
  line L671 (-80.5, 81.3301) -> (-83.5, 81.3301)
  line L672 (-83.5, 81.3301) -> (-85, 83.9282)
  line L673 (-85, 83.9282) -> (-83.5, 86.5263)
  line L674 (-83.5, 86.5263) -> (-80.5, 86.5263)
  line L675 (-72.5, 81.3301) -> (-75.5, 81.3301)
  line L676 (-75.5, 81.3301) -> (-77, 83.9282)
  line L677 (-80.5, 86.5263) -> (-79, 83.9282)
  line L678 (-77, 83.9282) -> (-75.5, 86.5263)
  line L679 (-71, 83.9282) -> (-72.5, 81.3301)
  line L680 (-75.5, 86.5263) -> (-72.5, 86.5263)
  line L681 (-72.5, 86.5263) -> (-71, 83.9282)
  line L682 (-79, 83.9282) -> (-80.5, 81.3301)
  line L683 (-51.5, 86.5263) -> (-48.5, 86.5263)
  line L684 (-48.5, 81.3301) -> (-51.5, 81.3301)
  line L685 (-51.5, 81.3301) -> (-53, 83.9282)
  line L686 (-53, 83.9282) -> (-51.5, 86.5263)
  line L687 (-56.5, 86.5263) -> (-55, 83.9282)
  line L688 (-55, 83.9282) -> (-56.5, 81.3301)
  line L689 (-56.5, 81.3301) -> (-59.5, 81.3301)
  line L690 (-59.5, 86.5263) -> (-56.5, 86.5263)
  line L691 (-61, 83.9282) -> (-59.5, 86.5263)
  line L692 (-64.5, 86.5263) -> (-63, 83.9282)
  line L693 (-63, 83.9282) -> (-64.5, 81.3301)
  line L694 (-67.5, 86.5263) -> (-64.5, 86.5263)
  line L695 (-64.5, 81.3301) -> (-67.5, 81.3301)
  line L696 (-69, 83.9282) -> (-67.5, 86.5263)
  line L697 (-67.5, 81.3301) -> (-69, 83.9282)
  line L698 (-59.5, 81.3301) -> (-61, 83.9282)
  line L699 (-76.5, 88.2583) -> (-79.5, 88.2583)
  line L700 (-79.5, 88.2583) -> (-81, 90.8564)
  line L701 (-79.5, 93.4545) -> (-76.5, 93.4545)
  line L702 (-81, 90.8564) -> (-79.5, 93.4545)
  line L703 (-39.5, 88.2583) -> (-41, 90.8564)
  line L704 (-41, 90.8564) -> (-39.5, 93.4545)
  line L705 (-43, 90.8564) -> (-44.5, 88.2583)
  line L706 (-44.5, 93.4545) -> (-43, 90.8564)
  line L707 (-47.5, 93.4545) -> (-44.5, 93.4545)
  line L708 (-49, 90.8564) -> (-47.5, 93.4545)
  line L709 (-47.5, 88.2583) -> (-49, 90.8564)
  line L710 (-52.5, 93.4545) -> (-51, 90.8564)
  line L711 (-51, 90.8564) -> (-52.5, 88.2583)
  line L712 (-55.5, 93.4545) -> (-52.5, 93.4545)
  line L713 (-52.5, 88.2583) -> (-55.5, 88.2583)
  line L714 (-44.5, 88.2583) -> (-47.5, 88.2583)
  line L715 (-57, 90.8564) -> (-55.5, 93.4545)
  line L716 (-60.5, 93.4545) -> (-59, 90.8564)
  line L717 (-59, 90.8564) -> (-60.5, 88.2583)
  line L718 (-63.5, 93.4545) -> (-60.5, 93.4545)
  line L719 (-60.5, 88.2583) -> (-63.5, 88.2583)
  line L720 (-63.5, 88.2583) -> (-65, 90.8564)
  line L721 (-65, 90.8564) -> (-63.5, 93.4545)
  line L722 (-55.5, 88.2583) -> (-57, 90.8564)
  line L723 (-67, 90.8564) -> (-68.5, 88.2583)
  line L724 (-68.5, 93.4545) -> (-67, 90.8564)
  line L725 (-68.5, 88.2583) -> (-71.5, 88.2583)
  line L726 (-71.5, 88.2583) -> (-73, 90.8564)
  line L727 (-73, 90.8564) -> (-71.5, 93.4545)
  line L728 (-75, 90.8564) -> (-76.5, 88.2583)
  line L729 (-76.5, 93.4545) -> (-75, 90.8564)
  line L730 (-71.5, 93.4545) -> (-68.5, 93.4545)
  line L731 (-47, 83.9282) -> (-48.5, 81.3301)
  line L732 (-48.5, 86.5263) -> (-47, 83.9282)
  line L733 (-45, 83.9282) -> (-43.5, 86.5263)
  line L734 (-43.5, 81.3301) -> (-45, 83.9282)
  line L735 (-43.5, 86.5263) -> (-40.5, 86.5263)
  line L736 (-40.5, 81.3301) -> (-43.5, 81.3301)
  line L737 (-40.5, 86.5263) -> (-39, 83.9282)
  line L738 (-39, 83.9282) -> (-40.5, 81.3301)
  line L739 (-11, 90.8564) -> (-12.5, 88.2583)
  line L740 (-12.5, 93.4545) -> (-11, 90.8564)
  line L741 (-24.5, 86.5263) -> (-23, 83.9282)
  line L742 (-23, 83.9282) -> (-24.5, 81.3301)
  line L743 (-27.5, 86.5263) -> (-24.5, 86.5263)
  line L744 (-24.5, 81.3301) -> (-27.5, 81.3301)
  line L745 (-29, 83.9282) -> (-27.5, 86.5263)
  line L746 (-27.5, 81.3301) -> (-29, 83.9282)
  line L747 (-31, 83.9282) -> (-32.5, 81.3301)
  line L748 (-32.5, 86.5263) -> (-31, 83.9282)
  line L749 (-32.5, 81.3301) -> (-35.5, 81.3301)
  line L750 (-35.5, 86.5263) -> (-32.5, 86.5263)
  line L751 (-35.5, 81.3301) -> (-37, 83.9282)
  line L752 (-37, 83.9282) -> (-35.5, 86.5263)
  line L753 (-19.5, 81.3301) -> (-21, 83.9282)
  line L754 (-21, 83.9282) -> (-19.5, 86.5263)
  line L755 (-19.5, 86.5263) -> (-16.5, 86.5263)
  line L756 (-16.5, 81.3301) -> (-19.5, 81.3301)
  line L757 (-16.5, 86.5263) -> (-15, 83.9282)
  line L758 (-15, 83.9282) -> (-16.5, 81.3301)
  line L759 (-20.5, 88.2583) -> (-23.5, 88.2583)
  line L760 (-23.5, 93.4545) -> (-20.5, 93.4545)
  line L761 (-19, 90.8564) -> (-20.5, 88.2583)
  line L762 (-20.5, 93.4545) -> (-19, 90.8564)
  line L763 (-17, 90.8564) -> (-15.5, 93.4545)
  line L764 (-15.5, 88.2583) -> (-17, 90.8564)
  line L765 (-12.5, 88.2583) -> (-15.5, 88.2583)
  line L766 (-15.5, 93.4545) -> (-12.5, 93.4545)
  line L767 (-25, 90.8564) -> (-23.5, 93.4545)
  line L768 (-28.5, 93.4545) -> (-27, 90.8564)
  line L769 (-27, 90.8564) -> (-28.5, 88.2583)
  line L770 (-31.5, 93.4545) -> (-28.5, 93.4545)
  line L771 (-28.5, 88.2583) -> (-31.5, 88.2583)
  line L772 (-33, 90.8564) -> (-31.5, 93.4545)
  line L773 (-31.5, 88.2583) -> (-33, 90.8564)
  line L774 (-23.5, 88.2583) -> (-25, 90.8564)
  line L775 (-36.5, 93.4545) -> (-35, 90.8564)
  line L776 (-35, 90.8564) -> (-36.5, 88.2583)
  line L777 (-39.5, 93.4545) -> (-36.5, 93.4545)
  line L778 (-36.5, 88.2583) -> (-39.5, 88.2583)
  line L779 (-13, 83.9282) -> (-11.5, 86.5263)
  line L780 (-8.5, 81.3301) -> (-11.5, 81.3301)
  line L781 (-11.5, 81.3301) -> (-13, 83.9282)
  line L782 (-8.5, 86.5263) -> (-7, 83.9282)
  line L783 (-7, 83.9282) -> (-8.5, 81.3301)
  line L784 (-4.5, 88.2583) -> (-7.5, 88.2583)
  line L785 (-7.5, 88.2583) -> (-9, 90.8564)
  line L786 (-3, 90.8564) -> (-4.5, 88.2583)
  line L787 (-4.5, 93.4545) -> (-3, 90.8564)
  line L788 (-7.5, 93.4545) -> (-4.5, 93.4545)
  line L789 (-9, 90.8564) -> (-7.5, 93.4545)
  line L790 (-11.5, 86.5263) -> (-8.5, 86.5263)
  line L791 (-3, 77) -> (-3, 90.8564) construction
  line L792 (-80.5, 95.3301) -> (-83.5, 95.3301)
  line L793 (-83.5, 95.3301) -> (-85, 97.9282)
  line L794 (-85, 97.9282) -> (-83.5, 100.5263)
  line L795 (-83.5, 100.5263) -> (-80.5, 100.5263)
  line L796 (-72.5, 95.3301) -> (-75.5, 95.3301)
  line L797 (-75.5, 95.3301) -> (-77, 97.9282)
  line L798 (-80.5, 100.5263) -> (-79, 97.9282)
  line L799 (-77, 97.9282) -> (-75.5, 100.5263)
  line L800 (-71, 97.9282) -> (-72.5, 95.3301)
  line L801 (-75.5, 100.5263) -> (-72.5, 100.5263)
  line L802 (-72.5, 100.5263) -> (-71, 97.9282)
  line L803 (-79, 97.9282) -> (-80.5, 95.3301)
  line L804 (-51.5, 100.5263) -> (-48.5, 100.5263)
  line L805 (-48.5, 95.3301) -> (-51.5, 95.3301)
  line L806 (-51.5, 95.3301) -> (-53, 97.9282)
  line L807 (-53, 97.9282) -> (-51.5, 100.5263)
  line L808 (-56.5, 100.5263) -> (-55, 97.9282)
  line L809 (-55, 97.9282) -> (-56.5, 95.3301)
  line L810 (-56.5, 95.3301) -> (-59.5, 95.3301)
  line L811 (-59.5, 100.5263) -> (-56.5, 100.5263)
  line L812 (-61, 97.9282) -> (-59.5, 100.5263)
  line L813 (-64.5, 100.5263) -> (-63, 97.9282)
  line L814 (-63, 97.9282) -> (-64.5, 95.3301)
  line L815 (-67.5, 100.5263) -> (-64.5, 100.5263)
  line L816 (-64.5, 95.3301) -> (-67.5, 95.3301)
  line L817 (-69, 97.9282) -> (-67.5, 100.5263)
  line L818 (-67.5, 95.3301) -> (-69, 97.9282)
  line L819 (-59.5, 95.3301) -> (-61, 97.9282)
  line L820 (-76.5, 102.2583) -> (-79.5, 102.2583)
  line L821 (-79.5, 102.2583) -> (-81, 104.8564)
  line L822 (-79.5, 107.4545) -> (-76.5, 107.4545)
  line L823 (-81, 104.8564) -> (-79.5, 107.4545)
  line L824 (-39.5, 102.2583) -> (-41, 104.8564)
  line L825 (-41, 104.8564) -> (-39.5, 107.4545)
  line L826 (-43, 104.8564) -> (-44.5, 102.2583)
  line L827 (-44.5, 107.4545) -> (-43, 104.8564)
  line L828 (-47.5, 107.4545) -> (-44.5, 107.4545)
  line L829 (-49, 104.8564) -> (-47.5, 107.4545)
  line L830 (-47.5, 102.2583) -> (-49, 104.8564)
  line L831 (-52.5, 107.4545) -> (-51, 104.8564)
  line L832 (-51, 104.8564) -> (-52.5, 102.2583)
  line L833 (-55.5, 107.4545) -> (-52.5, 107.4545)
  line L834 (-52.5, 102.2583) -> (-55.5, 102.2583)
  line L835 (-44.5, 102.2583) -> (-47.5, 102.2583)
  line L836 (-57, 104.8564) -> (-55.5, 107.4545)
  line L837 (-60.5, 107.4545) -> (-59, 104.8564)
  line L838 (-59, 104.8564) -> (-60.5, 102.2583)
  line L839 (-63.5, 107.4545) -> (-60.5, 107.4545)
  line L840 (-60.5, 102.2583) -> (-63.5, 102.2583)
  line L841 (-63.5, 102.2583) -> (-65, 104.8564)
  line L842 (-65, 104.8564) -> (-63.5, 107.4545)
  line L843 (-55.5, 102.2583) -> (-57, 104.8564)
  line L844 (-67, 104.8564) -> (-68.5, 102.2583)
  line L845 (-68.5, 107.4545) -> (-67, 104.8564)
  line L846 (-68.5, 102.2583) -> (-71.5, 102.2583)
  line L847 (-71.5, 102.2583) -> (-73, 104.8564)
  line L848 (-73, 104.8564) -> (-71.5, 107.4545)
  line L849 (-75, 104.8564) -> (-76.5, 102.2583)
  line L850 (-76.5, 107.4545) -> (-75, 104.8564)
  line L851 (-71.5, 107.4545) -> (-68.5, 107.4545)
  line L852 (-47, 97.9282) -> (-48.5, 95.3301)
  line L853 (-48.5, 100.5263) -> (-47, 97.9282)
  line L854 (-45, 97.9282) -> (-43.5, 100.5263)
  line L855 (-43.5, 95.3301) -> (-45, 97.9282)
  line L856 (-43.5, 100.5263) -> (-40.5, 100.5263)
  line L857 (-40.5, 95.3301) -> (-43.5, 95.3301)
  line L858 (-40.5, 100.5263) -> (-39, 97.9282)
  line L859 (-39, 97.9282) -> (-40.5, 95.3301)
  line L860 (-11, 104.8564) -> (-12.5, 102.2583)
  line L861 (-12.5, 107.4545) -> (-11, 104.8564)
  line L862 (-24.5, 100.5263) -> (-23, 97.9282)
  line L863 (-23, 97.9282) -> (-24.5, 95.3301)
  line L864 (-27.5, 100.5263) -> (-24.5, 100.5263)
  line L865 (-24.5, 95.3301) -> (-27.5, 95.3301)
  line L866 (-29, 97.9282) -> (-27.5, 100.5263)
  line L867 (-27.5, 95.3301) -> (-29, 97.9282)
  line L868 (-31, 97.9282) -> (-32.5, 95.3301)
  line L869 (-32.5, 100.5263) -> (-31, 97.9282)
  line L870 (-32.5, 95.3301) -> (-35.5, 95.3301)
  line L871 (-35.5, 100.5263) -> (-32.5, 100.5263)
  line L872 (-35.5, 95.3301) -> (-37, 97.9282)
  line L873 (-37, 97.9282) -> (-35.5, 100.5263)
  line L874 (-19.5, 95.3301) -> (-21, 97.9282)
  line L875 (-21, 97.9282) -> (-19.5, 100.5263)
  line L876 (-19.5, 100.5263) -> (-16.5, 100.5263)
  line L877 (-16.5, 95.3301) -> (-19.5, 95.3301)
  line L878 (-16.5, 100.5263) -> (-15, 97.9282)
  line L879 (-15, 97.9282) -> (-16.5, 95.3301)
  line L880 (-20.5, 102.2583) -> (-23.5, 102.2583)
  line L881 (-23.5, 107.4545) -> (-20.5, 107.4545)
  line L882 (-19, 104.8564) -> (-20.5, 102.2583)
  line L883 (-20.5, 107.4545) -> (-19, 104.8564)
  line L884 (-17, 104.8564) -> (-15.5, 107.4545)
  line L885 (-15.5, 102.2583) -> (-17, 104.8564)
  line L886 (-12.5, 102.2583) -> (-15.5, 102.2583)
  line L887 (-15.5, 107.4545) -> (-12.5, 107.4545)
  line L888 (-25, 104.8564) -> (-23.5, 107.4545)
  line L889 (-28.5, 107.4545) -> (-27, 104.8564)
  line L890 (-27, 104.8564) -> (-28.5, 102.2583)
  line L891 (-31.5, 107.4545) -> (-28.5, 107.4545)
  line L892 (-28.5, 102.2583) -> (-31.5, 102.2583)
  line L893 (-33, 104.8564) -> (-31.5, 107.4545)
  line L894 (-31.5, 102.2583) -> (-33, 104.8564)
  line L895 (-23.5, 102.2583) -> (-25, 104.8564)
  line L896 (-36.5, 107.4545) -> (-35, 104.8564)
  line L897 (-35, 104.8564) -> (-36.5, 102.2583)
  line L898 (-39.5, 107.4545) -> (-36.5, 107.4545)
  line L899 (-36.5, 102.2583) -> (-39.5, 102.2583)
  line L900 (-13, 97.9282) -> (-11.5, 100.5263)
  line L901 (-8.5, 95.3301) -> (-11.5, 95.3301)
  line L902 (-11.5, 95.3301) -> (-13, 97.9282)
  line L903 (-8.5, 100.5263) -> (-7, 97.9282)
  line L904 (-7, 97.9282) -> (-8.5, 95.3301)
  line L905 (-4.5, 102.2583) -> (-7.5, 102.2583)
  line L906 (-7.5, 102.2583) -> (-9, 104.8564)